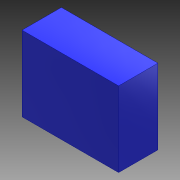
# Autodesk Inventor part: WR-LEN-base
Saved by Autodesk Inventor 2018 (Build 220112000, 112)
## iProperties
Created: 2022-04-20
Part Number: WR-LEN-base
Material: Generic
Document SubType Name: Modeling
Designer: pollak
Density: 1 g/cm^3
Appearance: Blue - Wall Paint - Glossy
Author: pollak
Autodesk Inventor part; units mm, degrees
ref_plane "YZ Plane" through (0, 0, 0) normal (1, 0, 0) x (0, 1, 0)
ref_plane "XZ Plane" through (0, 0, 0) normal (0, 1, 0) x (-1, 0, 0)
ref_plane "XY Plane" through (0, 0, 0) normal (0, 0, 1) x (1, 0, 0)
sketch "Sketch1" plane through (0, 0, 0) normal (0, 1, 0) x (-1, 0, 0)
  line L0 (67.5, 52.5) -> (-67.5, 52.5)
  line L1 (-67.5, 52.5) -> (-67.5, -52.5)
  line L2 (-67.5, -52.5) -> (67.5, -52.5)
  line L3 (67.5, -52.5) -> (67.5, 52.5)
  line L4 (67.5, 52.5) -> (-67.5, -52.5) construction
  line L5 (-67.5, 52.5) -> (67.5, -52.5) construction
  point P0 (0, 0)
  dimension "d0" = 135
  dimension "d1" = 105
  constraints: 12 end point, 2 midpoint, 2 parallel, 1 horizontal, 1 perpendicular
  measures "d0" distance of L2.end L1.end
  measures "d1" distance of L1.end L0.end
extrude "Extrusion1" add sketch "Sketch1" along normal blind 55
body "Solid1"
